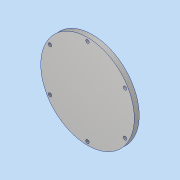
# Autodesk Inventor part: AluminumSealingDiscMidshipsMiddle
Saved by Autodesk Inventor 2017 (Build 210142000, 142)
## iProperties
Created: 2016-10-25
Part Number: AluminumSealingDiscMidshipsMiddle
Material: Aluminum 6061
Document SubType Name: Modeling
Designer: techn
Density: 2.7 g/cm^3
Appearance: Aluminum - Flat
Author: techn
Autodesk Inventor part; units mm, degrees
ref_plane "YZ Plane" through (0, 0, 0) normal (1, 0, 0) x (0, 1, 0)
ref_plane "XZ Plane" through (0, 0, 0) normal (0, 1, 0) x (-1, 0, 0)
ref_plane "XY Plane" through (0, 0, 0) normal (0, 0, 1) x (1, 0, 0)
sketch "Sketch1" plane through (0, 0, 0) normal (0, 0, 1) x (1, 0, 0)
  circle A0 centre (0, 0) radius 45.212
  dimension "d0" = 90.424
  constraints: 1 centre point, 1 coincident
  measures "d0" diameter of A0
extrude "Extrusion1" add sketch "Sketch1" along normal blind 4.7625
sketch "Sketch4" plane through (0, 0, 4.7625) normal (0, 0, 1) x (1, 0, 0)
  circle A0 centre (0, 41.91) radius 1.5875
  circle A1 centre (-36.2951, 20.955) radius 1.5875
  circle A2 centre (-36.2951, -20.955) radius 1.5875
  circle A3 centre (0, -41.91) radius 1.5875
  circle A4 centre (36.2951, -20.955) radius 1.5875
  circle A5 centre (36.2951, 20.955) radius 1.5875
  point P0 (0, 0)
  dimension "d14" = 3.175
  dimension "d15" = 41.91
  dimension "d18" = 360
  constraints: 6 centre point, 13 other
  measures "d14" diameter of A0
  measures "d15" distance of A0.centre point (0, 0)
extrude "Extrusion4" cut sketch "Sketch4" against normal blind 25.4
body "Solid1"
